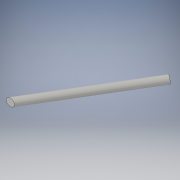
# Autodesk Inventor part: leg
Saved by Autodesk Inventor 2016 (Build 200138000, 138)
## iProperties
Created: 2019-01-25
Part Number: leg
Material: Generic
Document SubType Name: Modeling
Designer: Matthew Reese
Density: 1 g/cm^3
Appearance: Default
Author: Matthew Reese
Autodesk Inventor part; units mm, degrees
ref_plane "YZ Plane" through (0, 0, 0) normal (1, 0, 0) x (0, 1, 0)
ref_plane "XZ Plane" through (0, 0, 0) normal (0, 1, 0) x (-1, 0, 0)
ref_plane "XY Plane" through (0, 0, 0) normal (0, 0, 1) x (1, 0, 0)
sketch "Sketch2" plane through (0, 0, 0) normal (0, 1, 0) x (-1, 0, 0)
  line L0 (0, 0) -> (-152.5357, -253.8621)
  line L1 (-136.2067, -263.6736) -> (22.2244, 0)
  line L2 (-136.2067, -263.6736) -> (150.1458, -263.6736) construction
  line L3 (22.2244, 0) -> (0, 0)
  line L4 (-152.5357, -253.8621) -> (-136.2067, -263.6736)
  dimension "d9" = 296.164
  dimension "d12" = 59
  dimension "d13" = 19.05
  constraints: 11 end point, 1 horizontal, 1 perpendicular
  measures "d9" distance of L0.start L0.end
  measures "d12" angle of L2 L1
  measures "d13" distance between parallel lines of L0 L1
extrude "Extrusion1" add sketch "Sketch2" along normal blind 19.05
sketch "Sketch3" plane through (136.2067, 0, -263.6736) normal (0.5150381, 0, -0.8571673) x (-0.8571673, 0, -0.5150381)
  line L0 (0, 0) -> (0, 19.05) projected
  line L1 (0, 0) -> (-19.05, 0)
  line L2 (-19.05, 0) -> (-19.05, 19.05)
  line L3 (-19.05, 19.05) -> (0, 19.05)
  line L4 (0, 19.05) -> (0, 0)
  circle A0 centre (-9.525, 9.525) radius 9.525
  dimension "d18" = 19.05
  constraints: 8 end point, 2 parallel, 1 centre point, 1 horizontal, 1 perpendicular
  measures "d18" diameter of A0
extrude "Extrusion2" cut sketch "Sketch3" against normal through all contours L1 A0 L0 | A0 L3 L0 | L1 L2 A0 | A0 L2 L3
body "Solid1"
